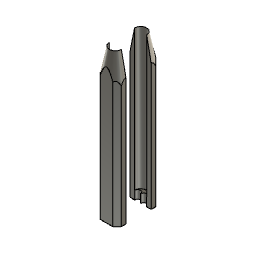
Badminton handle (without shaft connector) (Autodesk Fusion 360 design; units mm, degrees)
Autodesk Fusion 360 part; units mm, degrees
sketch "Sketch1" plane through (0, 0, 0) normal (0, 0, 1) x (1, 0, 0)
  line L0 (-15, 15) -> (10, 15)
  line L1 (10, 15) -> (10, -6)
  line L2 (10, -6) -> (-15, -6)
  line L3 (-15, -6) -> (-15, 15)
  dimension "d1" = 25
  dimension "d2" = 21
  constraint horizontal L0
  constraint vertical L1
  constraint horizontal L2
  constraint vertical L3
  measures "d1" distance of L0.start L0.end
  measures "d2" distance of L0.start L2.end
extrude "Extrude1" add sketch "Sketch1" along normal blind 190 makes body 1
chamfer "Chamfer1" distance 5 angle 45 4 edges at (10, -6, 95) (-15, -6, 95) (10, 15, 95) (-15, 15, 95) on bodies 1
sketch "Sketch2" plane through (0, 0, 0) normal (0, 0, 1) x (1, 0, 0)
sketch "Sketch3" plane through (0, 0, 190) normal (0, 0, 1) x (-1, 0, 0)
  line L0 (10, -15) -> (15, -10)
  line L1 (15, -10) -> (15, 1)
  line L2 (15, 1) -> (10, 6)
  line L3 (10, 6) -> (-5, 6)
  line L4 (-5, 6) -> (-10, 1)
  line L5 (-10, 1) -> (-10, -10)
  line L6 (-10, -10) -> (-5, -15)
  line L7 (-5, -15) -> (10, -15)
  circle A0 centre (2.5, -4.5) radius 3.6
  dimension "d7" = 7.2
  measures "d7" diameter of A0
extrude "Extrude2" cut sketch "Sketch3" against normal blind 120 contours A0 bodies 1
sketch "Sketch4" plane through (0, 0, 190) normal (0, 0, 1) x (-1, 0, 0)
  circle A0 centre (2.5, -4.5) radius 3.6
  line L0 (10, -15) -> (15, -10)
  line L1 (15, -10) -> (15, 1)
  line L2 (15, 1) -> (10, 6)
  line L3 (10, 6) -> (-5, 6)
  line L4 (-5, 6) -> (-10, 1)
  line L5 (-10, 1) -> (-10, -10)
  line L6 (-10, -10) -> (-5, -15)
  line L7 (-5, -15) -> (10, -15)
  circle A1 centre (2.5, -4.5) radius 7.15
  dimension "d19" = 14.3
  constraint concentric A0 A1
  measures "d19" diameter of A1
sketch "Sketch6" plane through (0, 0, 0) normal (0, 1, 0) x (1, 0, 0)
  line L0 (12.4931, -190, 4.5) -> (2, -190, 4.5)
  line L1 (2.0308, -190, 4.5) -> (14.8176, -126.8446, 4.5)
  line L2 (14.8176, -126.8446, 4.5) -> (12.4931, -190, 4.5)
revolve "Revolve1" cut sketch "Sketch6" angle 360 about axis through (-2.5, 4.5, 190) along (0, 0, 1) contours L0 L1 L2 in plane through (0, 4.5, 0) normal (0, 1, 0) bodies 1
sketch "Sketch7" plane through (0, 0, 0) normal (0, 0, -1) x (1, 0, 0)
  line L0 (-15, -10) -> (-10, -15)
  line L1 (-10, -15) -> (5, -15)
  line L2 (5, -15) -> (10, -10)
  line L3 (10, -10) -> (10, 1)
  line L4 (10, 1) -> (5, 6)
  line L5 (5, 6) -> (-10, 6)
  line L6 (-10, 6) -> (-15, 1)
  line L7 (-15, 1) -> (-15, -10)
  circle A0 centre (-6.09, -4.5) radius 3.5
  circle A1 centre (1.09, -4.5) radius 3.5
  line L8 (-6.09, -4.5) -> (-6.09, -15)
  line L9 (-6.09, -4.5) -> (-6.09, 6)
  line L10 (-6.09, -4.5) -> (1.09, -4.5)
  line L11 (-6.09, -4.5) -> (-15, -4.5)
  line L12 (1.09, -4.5) -> (10, -4.5)
  dimension "d15" = 7
  dimension "d16" = 7
  constraint coincident A0.centre L8.start
  constraint coincident L1 L8.end
  constraint perpendicular L1 L8
  constraint coincident L5 L9.end
  constraint perpendicular L5 L9
  constraint equal L8 L9
  constraint coincident A1.centre L10.end
  constraint horizontal L10
  constraint midpoint L7 L11.end
  constraint midpoint L3 L12.end
  constraint perpendicular L3 L12
  constraint equal L11 L12
  measures "d15" diameter of A0
  measures "d16" diameter of A1
extrude "Extrude3" cut sketch "Sketch7" against normal blind 190 contours A0 L8 L11 | A0 L9 L11 | A0 L8 L10 | A0 L9 L10 | A1 L10 L12 | A1 L10 L12 bodies 1
extrude "Extrude4" cut sketch "Sketch4" against normal blind 180 contours A0 | A1 bodies 1
ref_plane "WorkPlane1" through (-2.5, 4.5, 85.0888) normal (0, -1, 0) x (1, 0, 0)
split "Split1" by plane through (-2.5, 4.5, 85.0888) normal (0, -1, 0) bodies 1 makes body 2 at (-7.9772, -0.0959, 65.6879)
move_body "Move1" bodies 1 to x (1, 0, 0) y (0, 1, 0) z (0, 0, 1) at (0, 30, 0)
